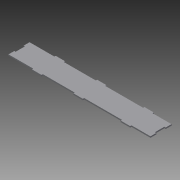
# Autodesk Inventor part: techo
Saved by Autodesk Inventor 2015 (Build 190159000, 159)
## iProperties
Created: 2017-09-28
Part Number: techo
Material: Generic
Document SubType Name: Modeling
Designer: Max
Density: 1 g/cm^3
Appearance: Default
Author: Max
Autodesk Inventor part; units mm, degrees
ref_plane "YZ Plane" through (0, 0, 0) normal (1, 0, 0) x (0, 1, 0)
ref_plane "XZ Plane" through (0, 0, 0) normal (0, 1, 0) x (-1, 0, 0)
ref_plane "XY Plane" through (0, 0, 0) normal (0, 0, 1) x (1, 0, 0)
sketch "Sketch1" plane through (0, 0, 0) normal (0, 0, 1) x (1, 0, 0)
  line L0 (0, 0) -> (600, 0)
  line L1 (600, 0) -> (600, 89)
  line L2 (600, 89) -> (0, 89)
  line L3 (0, 89) -> (0, 0)
  line L4 (105, 0) -> (145, 0)
  line L5 (145, 0) -> (145, -5.5)
  line L6 (145, -5.5) -> (105, -5.5)
  line L7 (105, -5.5) -> (105, 0)
  line L8 (280, 0) -> (320, 0)
  line L9 (320, 0) -> (320, -5.5)
  line L10 (320, -5.5) -> (280, -5.5)
  line L11 (280, -5.5) -> (280, 0)
  line L12 (480, 0) -> (520, 0)
  line L13 (520, 0) -> (520, -5.5)
  line L14 (520, -5.5) -> (480, -5.5)
  line L15 (480, -5.5) -> (480, 0)
  line L16 (105, 89) -> (145, 89)
  line L17 (145, 89) -> (145, 94.5)
  line L18 (145, 94.5) -> (105, 94.5)
  line L19 (105, 94.5) -> (105, 89)
  line L20 (280, 89) -> (320, 89)
  line L21 (320, 89) -> (320, 94.5)
  line L22 (320, 94.5) -> (280, 94.5)
  line L23 (280, 94.5) -> (280, 89)
  line L24 (480, 89) -> (520, 89)
  line L25 (520, 89) -> (520, 94.5)
  line L26 (520, 94.5) -> (480, 94.5)
  line L27 (480, 94.5) -> (480, 89)
  line L28 (0, 24.5) -> (5.5, 24.5)
  line L29 (5.5, 24.5) -> (5.5, 64.5)
  line L30 (5.5, 64.5) -> (0, 64.5)
  line L31 (0, 64.5) -> (0, 24.5)
  line L32 (600, 24.5) -> (594.5, 24.5)
  line L33 (594.5, 24.5) -> (594.5, 64.5)
  line L34 (594.5, 64.5) -> (600, 64.5)
  line L35 (600, 64.5) -> (600, 24.5)
  dimension "d0" = 600
  dimension "d1" = 89
  dimension "d2" = 40
  dimension "d3" = 5.5
  dimension "d4" = 40
  dimension "d5" = 5.5
  dimension "d6" = 40
  dimension "d7" = 5.5
  dimension "d8" = 5.5
  dimension "d9" = 40
  dimension "d10" = 5.5
  dimension "d11" = 40
  constraints: 72 end point, 12 parallel, 6 horizontal, 6 perpendicular, 5 point on line
  measures "d0" distance of L2.end L1.end
  measures "d1" distance of L1.end L0.end
  measures "d2" distance of L5.end L6.end
  measures "d3" distance of L4.end L5.end
  measures "d4" distance of L9.end L10.end
  measures "d5" distance of L8.end L9.end
  measures "d6" distance of L13.end L14.end
  measures "d7" distance of L12.end L13.end
  measures "d8" distance of L30.end L29.end
  measures "d9" distance of L29.end L28.end
  measures "d10" distance of L33.end L34.end
  measures "d11" distance of L32.end L33.end
extrude "Extrusion1" add sketch "Sketch1" along normal blind 5.5 contours L3 L28 L29 L30 L2 L1 L34 L33 L32 L0 | L0 L5 L6 L7 | L0 L9 L10 L11 | L19 L18 L17 L2 | L0 L13 L14 L15 | L23 L22 L21 L2 | L27 L26 L25 L2
body "Solid1"
